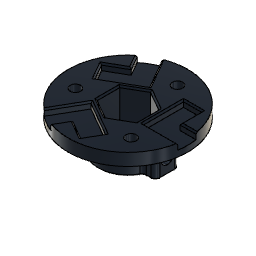
Picavet_supportgodethaut v9 (Autodesk Fusion 360 design; units mm, degrees)
Autodesk Fusion 360 part; units mm, degrees
sketch "Esquisse1" plane through (0, 0, 0) normal (0, 0, 1) x (1, 0, 0)
  circle A0 centre (0, 0) radius 20
  line L0 (19.7661, -3.05) -> (8.2661, -3.05)
  line L1 (8.2661, -3.05) -> (8.2661, 3.1)
  line L2 (14.3661, 3.05) -> (19.7661, 3.05)
  line L3 (8.2661, -3.05) -> (14.4602, -3.05)
  line L4 (14.3661, 10.35) -> (8.2661, 10.35)
  line L5 (8.2661, 10.35) -> (8.2661, -3.05)
  line L6 (0, 0) -> (29, 0) construction
  line L7 (14.3661, 3.05) -> (14.3661, 10.35)
  line L8 (-9.8244, 10.9164) -> (-16.1464, 7.2664)
  line L9 (-16.1464, 7.2664) -> (-13.0964, 1.9836)
  line L10 (-13.0964, 1.9836) -> (-1.4917, 8.6836)
  line L11 (-1.4917, 8.6836) -> (-4.5887, 14.0479)
  line L12 (-7.2417, 18.6429) -> (-1.4917, 8.6836)
  line L13 (-9.8244, 10.9164) -> (-12.5244, 15.5929)
  line L14 (-4.5417, -13.9664) -> (1.7803, -17.6164)
  line L15 (1.7803, -17.6164) -> (4.8303, -12.3336)
  line L16 (4.8303, -12.3336) -> (-6.7744, -5.6336)
  line L17 (-6.7744, -5.6336) -> (-9.8715, -10.9979)
  line L18 (-12.5244, -15.5929) -> (-6.7744, -5.6336)
  line L19 (-4.5417, -13.9664) -> (-7.2417, -18.6429)
  circle A1 centre (2.9108, 13.6941) radius 1.75
  line L20 (0, 0) -> (2.9108, 13.6941) construction
  circle A2 centre (-13.3148, -4.3262) radius 1.75
  circle A3 centre (10.404, -9.3678) radius 1.75
  line L21 (6.55, 3.7816) -> (0, 7.5633)
  line L22 (0, 7.5633) -> (-6.55, 3.7816)
  line L23 (-6.55, 3.7816) -> (-6.55, -3.7816)
  line L24 (-6.55, -3.7816) -> (0, -7.5633)
  line L25 (0, -7.5633) -> (6.55, -3.7816)
  line L26 (6.55, -3.7816) -> (6.55, 3.7816)
  dimension "d1" = 40
  dimension "d2" = 6.1
  dimension "d3" = 11.5
  dimension "d6" = 6.1
  dimension "d7" = 3.05
  dimension "d8" = 13.4
  dimension "d10" = 360
  dimension "d16" = 3.5
  dimension "d17" = 78
  dimension "d19" = 360
  dimension "d21" = 14
  dimension "d25" = 6.55
  constraint coincident A0.centre L6.start
  constraint horizontal L0
  constraint vertical L1
  constraint horizontal L2
  constraint coincident A0 L0.start
  constraint coincident A0 L2.end
  constraint horizontal L3
  constraint horizontal L4
  constraint vertical L5
  constraint horizontal L6
  constraint perpendicular L2 L7
  constraint coincident A1.centre L20.end
  constraint parallel L1 L26
  measures "d1" diameter of A0
  measures "d2" distance of L0.start L2.end
  measures "d3" distance of L0.start L0.end
  measures "d6" distance of L4.start L4.end
  measures "d7" distance of L2 L6
  measures "d8" distance of L0.end L4.end
  measures "d16" diameter of A1
  measures "d17" angle of L6 L20
  measures "d21" distance of A0.centre A1.centre
  measures "d25" distance of A0.centre L26
extrude "Extrusion1" add sketch "Esquisse1" against normal blind 4.1 contours A0 L0 L1 L2 L3 L4 L5 L7 | A0 L0 L1 L2 L3 L4 L5 L7 L8 L9 L10 L11 L12 L13 L14 L15 L16 L17 L18 L19 | A0 L8 L9 L10 L11 L12 L13 | A0 L14 L15 L16 L17 L18 L19 | A1 | A2 | A3 | L21 L22 L23 L24 L25 L26
extrude "Extrusion2" cut sketch "Esquisse1" against normal blind 2.1 contours A0 L0 L1 L2 L3 L4 L5 L7 | A0 L8 L9 L10 L11 L12 L13 | A0 L14 L15 L16 L17 L18 L19
chamfer "Chanfrein1" distance 0.5 angle 45 15 edges at (-4.3667, 13.6633, 0) (-11.1744, 13.2546, 0) (-12.9854, 9.0914, 0) (-14.6214, 4.625, 0) (-7.294, 5.3336, 0) (-9.6494, -10.6133, 0) (-0.972, -8.9836, 0) (-5.8917, -16.3046, 0) (-1.3807, -15.7914, 0) (3.3053, -14.975, 0) (8.2661, 3.65, 0) (14.0161, -3.05, 0) (17.0661, 3.05, 0) (14.3661, 6.7, 0) (11.3161, 10.35, 0)
extrude "Extrusion5" cut sketch "Esquisse1" against normal blind 4.1 contours A1 | A2 | A3
extrude "Extrusion6" cut sketch "Esquisse1" against normal blind 4.1 contours L21 L22 L23 L24 L25 L26
chamfer "Chanfrein4" distance 0.5 angle 45 6 edges at (-6.55, 0, 0) (-3.275, 5.6725, 0) (3.275, 5.6725, 0) (6.55, 0, 0) (3.275, -5.6725, 0) (-3.275, -5.6725, 0)
sketch "Esquisse2" plane through (0, 0, -4.1) normal (0, 0, -1) x (1, 0, 0)
  circle A0 centre (0, 0) radius 20
  circle A1 centre (2.9108, -13.6941) radius 1.75
  circle A2 centre (10.404, 9.3678) radius 1.75
  circle A3 centre (-13.3148, 4.3262) radius 1.75
  line L0 (9.1652, 4) -> (13.2, 4)
  line L1 (13.2, 4) -> (13.2, -4)
  line L2 (13.2, -4) -> (9.1652, -4)
  arc A4 (9.1652, 4) -> (9.1652, -4) centre (0, 0) ccw
  line L3 (6.55, -3.7816) -> (0, -7.5633)
  line L4 (0, -7.5633) -> (-6.55, -3.7816)
  line L5 (-6.55, -3.7816) -> (-6.55, 3.7816)
  line L6 (-6.55, 3.7816) -> (0, 7.5633)
  line L7 (0, 7.5633) -> (6.55, 3.7816)
  line L8 (6.55, 3.7816) -> (6.55, -3.7816)
  dimension "d36" = 20
  dimension "d37" = 8
  dimension "d39" = 4
  constraint concentric A0 A4
  constraint horizontal L0
  constraint vertical L1
  constraint horizontal L2
  measures "d36" diameter of A4
  measures "d37" distance of L0.end L1.end
  measures "d39" distance of A0.centre L2
extrude "Extrusion7" add sketch "Esquisse2" along normal blind 10 contours L0 L1 L2 A4
ref_plane "Plan de construction2" through (8.55, 0, -7.3) normal (-1, 0, 0) x (0, 1, 0)
sketch "Esquisse3" plane through (8.55, 0, 0) normal (-1, 0, 0) x (0, 1, 0)
  line L0 (4, -4.1) -> (-4, -4.1)
  line L1 (-4, -4.1) -> (-4, -14.1)
  line L2 (-4, -14.1) -> (4, -14.1)
  line L3 (4, -14.1) -> (4, -4.1)
  line L4 (-3, -14.1) -> (3, -14.1)
  line L5 (3, -14.1) -> (3, -9.1)
  line L6 (3, -9.1) -> (-3, -9.1) construction
  line L7 (-3, -9.1) -> (-3, -14.1)
  line L8 (3, -7.3679) -> (0, -5.6359)
  line L9 (0, -5.6359) -> (-3, -7.3679)
  line L10 (-3, -7.3679) -> (-3, -10.8321)
  line L11 (3, -10.8321) -> (3, -7.3679)
  line L12 (10.85, 0) -> (-3.55, 0)
  line L13 (3, 9.1) -> (-3, 9.1) construction
  line L14 (0, 5.6359) -> (-3, 7.3679)
  line L15 (3, 10.8321) -> (3, 7.3679)
  line L16 (-4, 14.1) -> (4, 14.1)
  line L17 (4, 4.1) -> (-4, 4.1)
  line L18 (-3, 14.1) -> (3, 14.1)
  line L19 (-3, 9.1) -> (-3, 14.1)
  line L20 (3, 14.1) -> (3, 9.1)
  line L21 (3, 7.3679) -> (0, 5.6359)
  line L22 (-4, 4.1) -> (-4, 14.1)
  line L23 (-3, 7.3679) -> (-3, 10.8321)
  line L24 (4, 14.1) -> (4, 4.1)
  point P0 (0, -9.1)
  point P1 (0, 9.1)
  dimension "d42" = 5
  dimension "d43" = 6
  dimension "d44" = 1
  constraint horizontal L4
  constraint vertical L5
  constraint horizontal L6
  constraint vertical L7
  constraint coincident L2 L4.start
  constraint midpoint L6 P0
  constraint symmetric L0.start L12 L17.start
  constraint symmetric L0.end L12 L17.end
  constraint symmetric L1.end L12 L16.start
  constraint symmetric L2.end L12 L16.end
  constraint symmetric L4.start L12 L18.start
  constraint symmetric L4.end L12 L18.end
  constraint symmetric L5.end L12 L13.start
  constraint symmetric L6.end L12 L13.end
  constraint symmetric L8.start L12 L15.end
  constraint symmetric L8.end L12 L14.start
  constraint symmetric L9.end L12 L14.end
  constraint symmetric L10.end L12 L23.end
  constraint symmetric L11.start L12 L15.start
  constraint symmetric P0 L12 P1
  measures "d42" distance of L4.end L5.end
  measures "d43" distance of L4.start L4.end
  measures "d44" distance of L2.end L4.end
extrude "Extrusion8" cut sketch "Esquisse3" against normal blind 2.4 contours L14 L15 L16 L18 L19 L20 L21 L23
hole "Perçage1" at (13.2, 0, -9.1) direction (-1, 0, 0) diameter 4 depth 7 tip angle 180
fillet "Congé1" radius 1.5 4 edges at (13.2, -4, -9.1) (13.2, 4, -9.1) (9.1652, 4, -9.1) (9.1652, -4, -9.1)
fillet "Congé2" radius 0.5 8 edges at (10.8998, -4, -14.1) (9.3334, -4.2104, -14.1) (-10, 0, -14.1) (9.3334, 4.2104, -14.1) (10.8998, 4, -14.1) (12.7607, 3.5607, -14.1) (13.2, 0, -14.1) (12.7607, -3.5607, -14.1)
equation "d6 = d2"
equation "d7 = d2 / 2"
equation "d39 = d37 / 2"
equation "d44 = ( 8 mm - d43 ) / 2"
